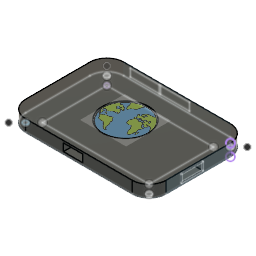
bottom panel (Autodesk Fusion 360 design; units mm, degrees)
part number: 2026-06-26-14-21-11-008
Autodesk Fusion 360 part; units mm, degrees
note: some values were not read from the file. Chosen so that the rebuilt part matches the saved one: the layout of a text. Set by a fixed rule: the direction of a hole.
sketch "Sketch1" plane through (0, 0, 0) normal (0, 1, 0) x (1, 0, 0)
  line L0 (0, 0) -> (63, 0)
  line L1 (63, 0) -> (63, -38)
  line L2 (63, -38) -> (0, -38)
  line L3 (0, -38) -> (0, 0)
  line L4 (0, 10) -> (63, 10)
  line L5 (73, 0) -> (73, -38)
  line L6 (63, -48) -> (0, -48)
  line L7 (-10, -38) -> (-10, 0)
  arc A0 (-10, -38) -> (0, -48) centre (0, -38) ccw
  arc A1 (63, -48) -> (73, -38) centre (63, -38) ccw
  arc A2 (0, 10) -> (-10, 0) centre (0, 0) ccw
  arc A3 (73, 0) -> (63, 10) centre (63, 0) ccw
  circle A4 centre (-5, -43) radius 1.45
  circle A5 centre (68, -43) radius 1.45
  circle A6 centre (68, 5) radius 1.45
  circle A7 centre (-5, 5) radius 1.45
  point P0 (-10, 10)
  point P1 (73, 10)
  point P2 (-10, -48)
  dimension "d1" = 63
  dimension "d2" = 38
  dimension "d3" = 83
  dimension "d4" = 58
  dimension "d5" = 10
  dimension "d6" = 10
  dimension "d7" = 10
  dimension "d8" = 10
  dimension "d9" = 10
  dimension "d42" = 2.9
  dimension "d43" = 5
  dimension "d44" = 2.9
  dimension "d45" = 5
  dimension "d46" = 5
  dimension "d47" = 2.9
  dimension "d48" = 5
  dimension "d49" = 5
  dimension "d50" = 2.9
  dimension "d51" = 5
  dimension "d52" = 5
  constraint horizontal L0
  constraint vertical L1
  constraint horizontal L2
  constraint vertical L3
  constraint coincident L0.start L3.end
  constraint horizontal L4
  constraint vertical L5
  constraint horizontal L6
  constraint vertical L7
  constraint coincident P2 L6
  constraint coincident P2 L7
  constraint tangent L6 A0
  constraint tangent L7 A0
  constraint tangent L5 A1
  constraint tangent L6 A1
  constraint equal A0 A1
  constraint coincident P0 L4
  constraint coincident P0 L7
  constraint tangent L4 A2
  constraint tangent L7 A2
  constraint coincident P1 L4
  constraint coincident P1 L5
  constraint tangent L4 A3
  constraint tangent L5 A3
  measures "d1" distance of L0.start L0.end
  measures "d2" distance of L0.start L2.end
  measures "d3" distance of P0 P1
  measures "d4" distance of P0 P2
  measures "d5" distance of L3 L7
  measures "d6" distance of L0 L4
  measures "d7" radius of A0
  measures "d8" radius of A2
  measures "d9" radius of A3
  measures "d42" diameter of A4
  measures "d43" distance of L6 A4.centre
  measures "d44" diameter of A5
  measures "d45" distance of L6 A5.centre
  measures "d46" distance of L5 A5.centre
  measures "d47" diameter of A6
  measures "d48" distance of L0 A6.centre
  measures "d49" distance of L5 A6.centre
  measures "d50" diameter of A7
  measures "d51" distance of L7 A7.centre
  measures "d52" distance of L4 A7.centre
extrude "Extrude1" add sketch "Sketch1" along normal blind 3 contours L0 L1 L2 L3
extrude "Extrude2" add sketch "Sketch1" along normal blind 3 contours L4 L5 L6 L7 A0 A1 A2 A3 | A4 | A5 | A6 | A7
extrude "Extrude3" add 1 faces at (21, 3, 28.6667) along direction (0, 1, 0) blind 4
extrude "Extrude4" cut sketch "Sketch1" along normal blind 6 contours L0 L1 L2 L3
sketch "Sketch3" plane through (0, 0, -10) normal (0, 0, -1) x (-1, 0, 0)
  line L0 (-63, 0) -> (0, 0)
  line L1 (0, 0) -> (0, 7)
  line L2 (0, 7) -> (-63, 7)
  line L3 (-63, 7) -> (-63, 0)
  line L4 (-3.9, 1.3) -> (-20.9, 1.3)
  line L5 (-20.9, 1.3) -> (-20.9, 5.8)
  line L6 (-20.9, 5.8) -> (-3.9, 5.8)
  line L7 (-3.9, 5.8) -> (-3.9, 1.3)
  line L8 (-21.8, 1.3) -> (-38.8, 1.3)
  line L9 (-38.8, 1.3) -> (-38.8, 5.8)
  line L10 (-38.8, 5.8) -> (-21.8, 5.8)
  line L11 (-21.8, 5.8) -> (-21.8, 1.3)
  dimension "d18" = 17
  dimension "d19" = 4.5
  dimension "d20" = 1.2
  dimension "d21" = 3.9
  dimension "d22" = 17
  dimension "d23" = 4.5
  dimension "d24" = 1.2
  dimension "d25" = 0.9
  constraint horizontal L4
  constraint vertical L5
  constraint horizontal L6
  constraint vertical L7
  constraint horizontal L8
  constraint vertical L9
  constraint horizontal L10
  constraint vertical L11
  measures "d18" distance of L4.start L4.end
  measures "d19" distance of L4.start L6.end
  measures "d20" distance of L2 L6
  measures "d21" distance of L1 L7
  measures "d22" distance of L8.start L8.end
  measures "d23" distance of L8.start L10.end
  measures "d24" distance of L2 L10
  measures "d25" distance of L5 L11
extrude "Extrude5" cut sketch "Sketch3" against normal blind 10 contours L4 L5 L6 L7
sketch "Sketch4" plane through (73, 0, 0) normal (1, 0, 0) x (0, 0, -1)
  line L0 (-38, 0) -> (0, 0)
  line L1 (0, 0) -> (0, 7)
  line L2 (0, 7) -> (-38, 7)
  line L3 (-38, 7) -> (-38, 0)
  line L4 (-16.5, 1.3) -> (-29, 1.3)
  line L5 (-29, 1.3) -> (-29, 5.8)
  line L6 (-29, 5.8) -> (-16.5, 5.8)
  line L7 (-16.5, 5.8) -> (-16.5, 1.3)
  line L8 (0, 0) -> (0, 7)
  dimension "d28" = 12.5
  dimension "d29" = 4.5
  dimension "d30" = 1.2
  dimension "d31" = 16.5
  constraint horizontal L4
  constraint vertical L5
  constraint horizontal L6
  constraint vertical L7
  measures "d28" distance of L4.start L4.end
  measures "d29" distance of L4.start L6.end
  measures "d30" distance of L2 L6
  measures "d31" distance of L7 L8
extrude "Extrude6" cut sketch "Sketch4" against normal blind 10 contours L4 L5 L6 L7
sketch "Sketch5" plane through (0, 0, 48) normal (0, 0, 1) x (1, 0, 0)
  line L0 (0, 0) -> (63, 0)
  line L1 (63, 0) -> (63, 7)
  line L2 (63, 7) -> (0, 7)
  line L3 (0, 7) -> (0, 0)
  line L4 (33.7, 1.3) -> (22.3, 1.3)
  line L5 (22.3, 1.3) -> (22.3, 5.8)
  line L6 (22.3, 5.8) -> (33.7, 5.8)
  line L7 (33.7, 5.8) -> (33.7, 1.3)
  dimension "d34" = 11.4
  dimension "d35" = 4.5
  dimension "d36" = 1.2
  dimension "d37" = 29.3
  constraint horizontal L4
  constraint vertical L5
  constraint horizontal L6
  constraint vertical L7
  measures "d34" distance of L4.start L4.end
  measures "d35" distance of L4.start L6.end
  measures "d36" distance of L2 L6
  measures "d37" distance of L1 L7
extrude "Extrude7" cut sketch "Sketch3" against normal blind 10 contours L8 L9 L10 L11
extrude "Extrude8" cut sketch "Sketch5" against normal blind 10 contours L4 L5 L6 L7
hole "Hole1" at (-5, 0, 43) direction (0, 1, 0) diameter 2.9 depth 6 tip angle 118
hole "Hole2" at (-5, 0, -5) direction (0, 1, 0) diameter 2.9 depth 6 tip angle 118
hole "Hole3" at (68, 0, -5) direction (0, 1, 0) diameter 2.9 depth 6 tip angle 118
hole "Hole4" at (68, 0, 43) direction (0, 1, 0) diameter 2.9 depth 6 tip angle 118
sketch "Sketch6" plane through (-10, 0, 0) normal (-1, 0, 0) x (0, 0, 1)
  line L0 (0, 0) -> (38, 0)
  line L1 (38, 0) -> (38, 7)
  line L2 (38, 7) -> (0, 7)
  line L3 (0, 7) -> (0, 0)
  line L4 (28.7985, 5.679) -> (15.4233, 5.679) construction
  line L5 (15.4233, 5.679) -> (15.4233, 2.4826) construction
  line L6 (15.4233, 2.4826) -> (28.7985, 2.4826) construction
  line L7 (28.7985, 2.4826) -> (28.7985, 5.679) construction
  line L8 (18.1232, 7) -> (7, 7) construction
  line L9 (7, 7) -> (7, 2.3654) construction
  line L10 (7, 2.3654) -> (18.1232, 2.3654) construction
  line L11 (18.1232, 2.3654) -> (18.1232, 7) construction
  dimension "d65" = 2.5
  dimension "d67" = 2.5
  text T0 "Travel " font "Arial" height 2.5 align left top in box 13.3752 x 3.1964 at (28.7985, 5.679) x (-1, 0) y (0, -1) spacing 1 kerned
  text T1 "Usb-Hub" font "Arial" height 2.5 align left top in box 11.1232 x 4.6346 at (18.1232, 7) x (-1, 0) y (0, -1) spacing 1
extrude "Extrude9" cut sketch "Sketch6" against normal blind 0.3 text T0
extrude "Extrude10" cut sketch "Sketch6" against normal blind 0.3 text T1
sketch "Sketch7" plane through (0, 7, 0) normal (0, 1, 0) x (-1, 0, 0)
  arc A0 (-63, 48) -> (-73, 38) centre (-63, 38) ccw
  line L0 (-73, 38) -> (-73, 0)
  arc A1 (-73, 0) -> (-63, -10) centre (-63, 0) ccw
  line L1 (-63, -10) -> (0, -10)
  arc A2 (0, -10) -> (10, 0) centre (0, 0) ccw
  line L2 (10, 0) -> (10, 38)
  arc A3 (10, 38) -> (0, 48) centre (0, 38) ccw
  line L3 (0, 48) -> (-63, 48)
  circle A4 centre (-30, 19) radius 13.6015
extrude "Extrude11" cut sketch "Sketch7" against normal blind 0.3 contours A4
equation "d66 = 'Travel '"
equation "d68 = 'Usb-Hub'"
